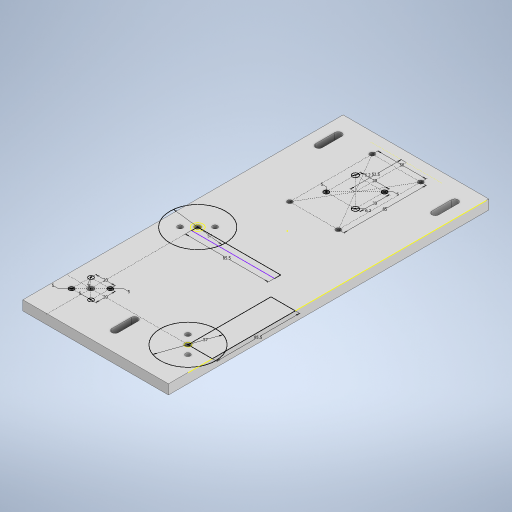
# Autodesk Inventor part: Base
Saved by Autodesk Inventor 2024 (Build 280153000, 153)
## iProperties
Created: 2026-02-25
Part Number: Base
Material: Generic
Document SubType Name: Modeling
Designer: Nathan
Density: 1 g/cm^3
Appearance: Default
Author: Nathan
Autodesk Inventor part; units mm, degrees
ref_plane "YZ Plane" through (0, 0, 0) normal (1, 0, 0) x (0, 1, 0)
ref_plane "XZ Plane" through (0, 0, 0) normal (0, 1, 0) x (-1, 0, 0)
ref_plane "XY Plane" through (0, 0, 0) normal (0, 0, 1) x (1, 0, 0)
sketch "Sketch1" plane through (0, 0, 0) normal (0, 1, 0) x (-1, 0, 0)
  line L0 (90, 130) -> (-90, 130)
  line L1 (-90, 130) -> (-90, -130)
  line L2 (-90, -130) -> (90, -130)
  line L3 (90, -130) -> (90, 130)
  line L4 (90, 130) -> (-90, -130) construction
  line L5 (-90, 130) -> (90, -130) construction
  point P0 (0, 0)
  dimension "d0" = 180
  dimension "d1" = 260
  constraints: 12 end point, 2 midpoint, 2 parallel, 1 horizontal, 1 perpendicular
  measures "d0" distance of L2.end L1.end
  measures "d1" distance of L1.end L0.end
extrude "Extrusion1" add sketch "Sketch1" along normal blind 10
sketch "Sketch2" plane through (0, 10, 0) normal (0, 1, 0) x (1, 0, 0)
  line L0 (90, 130) -> (-90, 130) construction
  line L1 (0, 130) -> (0, 120) construction
  line L2 (0, 130) -> (10, 130) construction
  line L3 (0, 120) -> (0, 70) construction
  line L4 (-37.5, 17.5) -> (37.5, 17.5)
  line L5 (37.5, 17.5) -> (37.5, 122.5)
  line L6 (37.5, 122.5) -> (-37.5, 122.5)
  line L7 (-37.5, 122.5) -> (-37.5, 17.5)
  line L8 (-37.5, 17.5) -> (37.5, 122.5) construction
  line L9 (37.5, 17.5) -> (-37.5, 122.5) construction
  point P0 (0, 0)
  dimension "d4" = 10
  dimension "d6" = 50
  dimension "d7" = 75
  dimension "d8" = 105
  constraints: 18 end point, 3 midpoint, 3 perpendicular, 2 horizontal, 2 parallel, 1 vertical
  measures "d4" distance of L1.start L1.end
  measures "d6" distance of L1.end L3.end
  measures "d7" distance of L6.end L5.end
  measures "d8" distance of L5.end L4.end
extrude "Extrusion2" cut sketch "Sketch2" against normal blind 2
sketch "Sketch3" plane through (0, 8, 0) normal (0, 1, 0) x (1, 0, 0)
  line L0 (-37.5, 122.5) -> (37.5, 122.5) construction
  line L1 (0, 122.5) -> (0, 70) construction
  line L2 (-15, 55) -> (15, 55) construction
  line L3 (15, 55) -> (15, 85) construction
  line L4 (15, 85) -> (-15, 85) construction
  line L5 (-15, 85) -> (-15, 55) construction
  line L6 (-15, 55) -> (15, 85) construction
  line L7 (15, 55) -> (-15, 85) construction
  circle A0 centre (15, 55) radius 3.1
  circle A1 centre (-15, 85) radius 3.1
  line L8 (-25, 27.5) -> (25, 27.5) construction
  line L9 (25, 27.5) -> (25, 112.5) construction
  line L10 (25, 112.5) -> (-25, 112.5) construction
  line L11 (-25, 112.5) -> (-25, 27.5) construction
  line L12 (-25, 27.5) -> (25, 112.5) construction
  line L13 (25, 27.5) -> (-25, 112.5) construction
  circle A2 centre (-15, 55) radius 2.5
  circle A3 centre (15, 85) radius 2.5
  point P0 (0, 0)
  dimension "d11" = 52.5
  dimension "d12" = 30
  dimension "d13" = 30
  dimension "d14" = 6.2
  dimension "d15" = 6.2
  dimension "d19" = 50
  dimension "d20" = 85
  dimension "d175" = 5
  dimension "d176" = 5
  constraints: 26 end point, 5 midpoint, 4 centre point, 4 coincident, 4 parallel, 2 horizontal, 2 perpendicular, 1 vertical
  measures "d11" distance of L1.start L1.end
  measures "d12" distance of L4.end L3.end
  measures "d13" distance of L3.end L2.end
  measures "d14" diameter of A0
  measures "d15" diameter of A1
  measures "d19" distance of L10.end L9.end
  measures "d20" distance of L9.end L8.end
  measures "d175" diameter of A2
  measures "d176" diameter of A3
extrude "Extrusion3" cut sketch "Sketch3" against normal blind 6 contours A2 | A3
hole "Hole1" at (-25, 8, -27.5) at (25, 8, -27.5) at (25, 8, -112.5) at (-25, 8, -112.5) direction (0, -1, 0) diameter 4.917 depth 10 thread size "M6x1" class "6H" standard "ANSI Metric M Profile"
sketch "Sketch6" plane through (0, 10, 0) normal (0, 1, 0) x (1, 0, 0)
  line L0 (90, -130) -> (90, 130) projected
  line L1 (90, -130) -> (-90, -130)
  line L2 (-90, -130) -> (-90, -192.5)
  line L3 (-90, -192.5) -> (90, -192.5)
  line L4 (90, -192.5) -> (90, -130)
  point P0 (0, 0)
  dimension "d101" = 62.5
  constraints: 8 end point, 2 parallel, 1 horizontal, 1 perpendicular
  measures "d101" distance of L2.end L1.end
extrude "Extrusion15" add sketch "Sketch6" against normal blind 10
sketch "Sketch13" plane through (0, 10, 0) normal (0, 1, 0) x (1, 0, 0)
  line L0 (90, -192.5) -> (-90, -192.5) construction
  line L1 (90, -192.5) -> (50, -192.5) construction
  line L2 (50, -192.5) -> (50, -152.5) construction
  line L3 (50, -152.5) -> (90, -152.5) construction
  line L4 (90, -152.5) -> (90, -192.5) construction
  line L5 (-90, 130) -> (-90, -192.5) construction
  line L6 (-90, -192.5) -> (-50, -192.5) construction
  line L7 (-50, -192.5) -> (-50, -42.5) construction
  line L8 (-50, -42.5) -> (-90, -42.5) construction
  line L9 (-90, -42.5) -> (-90, -192.5) construction
  line L10 (32, -170.5) -> (68, -170.5)
  line L11 (68, -170.5) -> (68, -134.5)
  line L12 (68, -134.5) -> (32, -134.5)
  line L13 (32, -134.5) -> (32, -170.5)
  line L14 (32, -170.5) -> (68, -134.5) construction
  line L15 (68, -170.5) -> (32, -134.5) construction
  line L16 (-68, -60.5) -> (-32, -60.5)
  line L17 (-32, -60.5) -> (-32, -24.5)
  line L18 (-32, -24.5) -> (-68, -24.5)
  line L19 (-68, -24.5) -> (-68, -60.5)
  line L20 (-68, -60.5) -> (-32, -24.5) construction
  line L21 (-32, -60.5) -> (-68, -24.5) construction
  point P0 (0, 0)
  dimension "d104" = 40
  dimension "d105" = 40
  dimension "d106" = 40
  dimension "d107" = 150
  dimension "d108" = 36
  dimension "d109" = 36
  dimension "d110" = 36
  dimension "d111" = 36
  constraints: 40 end point, 8 parallel, 4 horizontal, 4 midpoint, 4 perpendicular
  measures "d104" distance of L2.end L3.end
  measures "d105" distance of L1.end L2.end
  measures "d106" distance of L8.end L7.end
  measures "d107" distance of L7.end L6.end
  measures "d108" distance of L12.end L11.end
  measures "d109" distance of L11.end L10.end
  measures "d110" distance of L18.end L17.end
  measures "d111" distance of L17.end L16.end
extrude "Extrusion16" cut sketch "Sketch13" against normal blind 2
sketch "Sketch14" plane through (0, 8, 0) normal (0, 1, 0) x (1, 0, 0)
  line L0 (68, -170.5) -> (32, -170.5) construction
  line L1 (68, -170.5) -> (32, -134.5) construction
  line L2 (68, -134.5) -> (68, -170.5) construction
  line L3 (68, -134.5) -> (32, -170.5) construction
  line L4 (-32, -24.5) -> (-32, -60.5) construction
  line L5 (-32, -60.5) -> (-68, -24.5) construction
  line L6 (-68, -24.5) -> (-32, -24.5) construction
  line L7 (-32, -60.5) -> (-68, -60.5) construction
  line L8 (-32, -24.5) -> (-68, -60.5) construction
  line L9 (50, -152.5) -> (50, -134.5) construction
  line L10 (32, -134.5) -> (68, -134.5) construction
  line L11 (-50, -42.5) -> (-50, -24.5) construction
  line L12 (41, -161.5) -> (59, -161.5) construction
  line L13 (59, -161.5) -> (59, -143.5) construction
  line L14 (59, -143.5) -> (41, -143.5) construction
  line L15 (41, -143.5) -> (41, -161.5) construction
  line L16 (41, -161.5) -> (59, -143.5) construction
  line L17 (59, -161.5) -> (41, -143.5) construction
  line L18 (-59, -51.5) -> (-41, -51.5) construction
  line L19 (-41, -51.5) -> (-41, -33.5) construction
  line L20 (-41, -33.5) -> (-59, -33.5) construction
  line L21 (-59, -33.5) -> (-59, -51.5) construction
  line L22 (-59, -51.5) -> (-41, -33.5) construction
  line L23 (-41, -51.5) -> (-59, -33.5) construction
  circle A0 centre (59, -161.5) radius 2.5
  circle A1 centre (41, -143.5) radius 2.5
  circle A2 centre (-59, -51.5) radius 2.5
  circle A3 centre (-41, -33.5) radius 2.5
  point P0 (0, 0)
  dimension "d121" = 18
  dimension "d122" = 18
  dimension "d123" = 18
  dimension "d124" = 18
  dimension "d125" = 5
  dimension "d126" = 5
  dimension "d127" = 5
  dimension "d128" = 5
  constraints: 36 end point, 8 midpoint, 4 centre point, 4 coincident, 4 parallel, 3 perpendicular, 2 horizontal
  measures "d121" distance of L14.end L13.end
  measures "d122" distance of L13.end L12.end
  measures "d123" distance of L20.end L19.end
  measures "d124" distance of L19.end L18.end
  measures "d125" diameter of A0
  measures "d126" diameter of A1
  measures "d127" diameter of A2
  measures "d128" diameter of A3
sketch "Sketch15" plane through (0, 0, 0) normal (0, -1, 0) x (1, 0, 0)
  line L0 (68, 134.5) -> (68, 170.5) construction
  line L1 (68, 170.5) -> (32, 134.5) construction
  line L2 (32, 134.5) -> (68, 134.5) construction
  line L3 (68, 134.5) -> (32, 170.5) construction
  line L4 (32, 170.5) -> (50, 152.5) construction
  line L5 (-32, 24.5) -> (-32, 60.5) construction
  line L6 (-32, 60.5) -> (-68, 24.5) construction
  line L7 (-68, 24.5) -> (-32, 24.5) construction
  line L8 (-32, 24.5) -> (-68, 60.5) construction
  line L9 (-68, 60.5) -> (-50, 42.5) construction
  point P0 (0, 0)
  constraints: 15 end point, 2 midpoint, 2 perpendicular
extrude "Extrusion17" cut sketch "Sketch14" against normal blind 6
sketch "Sketch16" plane through (0, 10, 0) normal (0, 1, 0) x (1, 0, 0)
  line L0 (32, -170.5) -> (32, -134.5) construction
  line L1 (32, -134.5) -> (-90, -134.5) construction
  line L2 (-90, 130) -> (-90, -192.5) construction
  line L3 (32, -170.5) -> (-90, -170.5) construction
  line L4 (-32, -60.5) -> (-68, -60.5) construction
  line L5 (-32, -60.5) -> (-32, -134.5) construction
  line L6 (-32, -134.5) -> (-63, -134.5)
  line L7 (-63, -134.5) -> (-63, -165.5)
  line L8 (-63, -165.5) -> (-32, -165.5)
  line L9 (-32, -165.5) -> (-32, -134.5)
  point P0 (0, 0)
  dimension "d140" = 31
  dimension "d141" = 31
  constraints: 14 end point, 3 horizontal, 2 parallel, 2 point on line, 1 perpendicular, 1 vertical
  measures "d140" distance of L8.end L7.end
  measures "d141" distance of L7.end L6.end
extrude "Extrusion18" cut sketch "Sketch16" against normal blind 2
sketch "Sketch18" plane through (0, 0, 0) normal (0, -1, 0) x (1, 0, 0)
  line L0 (-90, 192.5) -> (90, 192.5) projected
  line L1 (-90, -130) -> (-90, 192.5) projected
  line L2 (90, 192.5) -> (-90, 192.5)
  line L3 (-90, 192.5) -> (-90, -130)
  line L4 (-90, -130) -> (90, -130)
  line L5 (90, -130) -> (90, 192.5)
  point P0 (0, 0)
  constraints: 8 end point, 2 parallel, 1 horizontal, 1 perpendicular
extrude "Extrusion20" add sketch "Sketch18" along normal blind 2
sketch "Sketch19" plane through (0, -2, 0) normal (0, -1, 0) x (1, 0, 0)
  circle A0 centre (50, 152.5) radius 2.4585 construction
  circle A1 centre (-50, 42.5) radius 2.4585 construction
  line L0 (50, 152.5) -> (-50, 42.5) construction
  line L1 (-32, 165.5) -> (-63, 165.5) construction
  line L2 (-32, 134.5) -> (-32, 165.5) construction
  line L3 (-63, 165.5) -> (-32, 134.5) construction
  line L4 (-63, 134.5) -> (-32, 134.5) construction
  line L5 (-63, 134.5) -> (-32, 165.5) construction
  line L6 (-47.5, 150) -> (-32, 150) construction
  point P0 (0, 0)
  constraints: 8 end point, 2 midpoint
hole "Hole6" at (-50, -2, 42.5) at (50, -2, 152.5) direction (0, 1, 0) diameter 6.1 end through all countersink diameter 11 countersink angle 90 clearance for "Countersunk Flat Head Screw ISO 2009/7046" size "M6" standard "ISO"
sketch "Sketch20" plane through (0, 10, 0) normal (0, 1, 0) x (1, 0, 0)
  line L0 (-90, 130) -> (90, 130) construction
  line L1 (-90, -192.5) -> (-90, 130) construction
  line L2 (90, 130) -> (-90, 130) construction
  line L3 (-90, 130) -> (-90, -192.5) construction
  line L4 (-90, -192.5) -> (90, -192.5) construction
  line L5 (90, -192.5) -> (90, 130) construction
  line L6 (-90, -192.5) -> (-75, -192.5)
  line L7 (-75, -177.5) -> (-75, 130)
  line L8 (-75, 130) -> (-90, 130)
  line L9 (-90, 130) -> (-90, -192.5)
  line L10 (90, 130) -> (75, 130)
  line L11 (75, 130) -> (75, -177.5)
  line L12 (75, -192.5) -> (90, -192.5)
  line L13 (90, -192.5) -> (90, 130)
  line L14 (90, -192.5) -> (-90, -192.5)
  line L15 (-90, -192.5) -> (-90, -177.5)
  line L16 (-75, -177.5) -> (75, -177.5)
  line L17 (90, -177.5) -> (90, -192.5)
  point P0 (0, 0)
  dimension "d166" = 180
  dimension "d167" = 15
  dimension "d168" = 15
  dimension "d169" = 15
  constraints: 32 end point, 8 parallel, 4 horizontal, 4 perpendicular, 3 point on line
  measures "d166" distance of L4.end L1.start
  measures "d167" distance of L8.end L7.end
  measures "d168" distance of L12.end L12.start
  measures "d169" distance of L14.end L15.end
extrude "Extrusion21" cut sketch "Sketch20" against normal through all
sketch "Sketch21" plane through (0, 10, 0) normal (0, 1, 0) x (1, 0, 0)
  line L0 (-75, -177.5) -> (-75, 130) projected
  line L1 (75, 130) -> (75, -177.5) projected
  line L2 (-75, -177.5) -> (75, -177.5)
  line L3 (75, -177.5) -> (75, 130)
  line L4 (75, 130) -> (-75, 130)
  line L5 (-75, 130) -> (-75, -177.5)
  point P0 (0, 0)
  constraints: 8 end point, 2 parallel, 1 horizontal, 1 perpendicular
extrude "Extrusion22" cut sketch "Sketch21" against normal blind 2
sketch "Sketch22" plane through (0, 8, 0) normal (0, 1, 0) x (1, 0, 0)
  circle A0 centre (-50, -42.5) radius 3.05 projected
  circle A1 centre (-50, -42.5) radius 28.5
  circle A2 centre (50, -152.5) radius 3.05 projected
  circle A3 centre (50, -152.5) radius 28.5
  line L0 (75, 130) -> (75, -177.5) projected
  line L1 (50, -152.5) -> (75, -152.5)
  line L2 (75, -152.5) -> (75, -67)
  line L3 (75, -67) -> (50, -67)
  line L4 (50, -67) -> (50, -152.5)
  circle A4 centre (-50, -42.5) radius 5.5 projected
  line L5 (-50, -42.5) -> (35.5, -42.5)
  line L6 (35.5, -42.5) -> (35.5, -48.8)
  line L7 (35.5, -48.8) -> (-50, -48.8)
  line L8 (-50, -48.8) -> (-50, -42.5)
  point P0 (0, 0)
  dimension "d182" = 57
  dimension "d183" = 57
  dimension "d184" = 85.5
  dimension "d185" = 85.5
  constraints: 16 end point, 4 parallel, 2 centre point, 2 coincident, 2 horizontal, 2 perpendicular, 1 point on line
  measures "d182" diameter of A1
  measures "d183" diameter of A3
  measures "d184" distance of L2.end L1.end
  measures "d185" distance of L6.end L7.end
sketch "Sketch23" plane through (0, 8, 0) normal (0, 1, 0) x (1, 0, 0)
  line L0 (75, 130) -> (75, -177.5) projected
  line L1 (-75, -177.5) -> (-75, 130) projected
  line L2 (75, 130) -> (-75, 130)
  line L3 (-75, 130) -> (-75, -177.5)
  line L4 (-75, -177.5) -> (75, -177.5)
  line L5 (75, -177.5) -> (75, 130)
  line L6 (-75, 130) -> (75, 130) projected
  line L7 (75, 130) -> (-75, 130)
  line L8 (-75, 130) -> (-75, 132.5)
  line L9 (-75, 132.5) -> (75, 132.5)
  line L10 (75, 132.5) -> (75, 130)
  line L11 (-75, -177.5) -> (75, -177.5)
  line L12 (75, -177.5) -> (75, -197.5)
  line L13 (75, -197.5) -> (-75, -197.5)
  line L14 (-75, -197.5) -> (-75, -177.5)
  point P0 (0, 0)
  dimension "d186" = 2.5
  dimension "d187" = 20
  constraints: 24 end point, 6 parallel, 3 horizontal, 3 perpendicular
  measures "d186" distance of L7.end L8.end
  measures "d187" distance of L11.end L12.end
extrude "Extrusion23" add sketch "Sketch23" against normal blind 10 contours L2 L8 L9 L10 | L12 L13 L14 L4
sketch "Sketch24" plane through (0, 8, 0) normal (0, 1, 0) x (1, 0, 0)
  circle A0 centre (50, -152.5) radius 3.05 construction
  line L0 (50, -152.5) -> (-74.625, -152.5) construction
  circle A1 centre (-50, -42.5) radius 3.05 construction
  line L1 (-50, -42.5) -> (-50, -199.1809) construction
  line L2 (-60, -162.5) -> (-40, -162.5) construction
  line L3 (-40, -162.5) -> (-40, -142.5) construction
  line L4 (-40, -142.5) -> (-60, -142.5) construction
  line L5 (-60, -142.5) -> (-60, -162.5) construction
  line L6 (-60, -162.5) -> (-40, -142.5) construction
  line L7 (-40, -162.5) -> (-60, -142.5) construction
  circle A2 centre (-60, -162.5) radius 2.5
  circle A3 centre (-40, -142.5) radius 2.5
  circle A4 centre (-40, -162.5) radius 2.5
  circle A5 centre (-60, -142.5) radius 2.5
  point P0 (0, 0)
  point P1 (-50, -152.5)
  dimension "d190" = 20
  dimension "d191" = 20
  dimension "d192" = 5
  dimension "d193" = 5
  dimension "d221" = 5
  dimension "d222" = 5
  constraints: 16 end point, 4 centre point, 4 coincident, 2 horizontal, 2 midpoint, 2 parallel, 2 perpendicular, 2 point on line
  measures "d190" distance of L4.end L3.end
  measures "d191" distance of L3.end L2.end
  measures "d192" diameter of A2
  measures "d193" diameter of A3
  measures "d221" diameter of A4
  measures "d222" diameter of A5
extrude "Extrusion24" cut sketch "Sketch24" against normal blind 6 contours A2 | A3
sketch "Sketch25" plane through (0, -2, 0) normal (0, -1, 0) x (1, 0, 0)
  circle A0 centre (50, 152.5) radius 3.05 construction
  line L0 (50, 152.5) -> (-75, 152.5) construction
  line L1 (-75, 197.5) -> (-75, -132.5) construction
  circle A1 centre (-50, 42.5) radius 3.05 construction
  line L2 (-50, 42.5) -> (-50, 197.5) construction
  line L3 (75, 197.5) -> (-75, 197.5) construction
  circle A2 centre (-50, 152.5) radius 7.5 construction
  point P0 (0, 0)
  dimension "d213" = 15
  constraints: 4 end point, 4 point on line, 1 centre point, 1 horizontal, 1 perpendicular
  measures "d213" diameter of A2
hole "Hole10" at (-50, -2, 152.5) direction (0, 1, 0) diameter 6.1 end through all countersink diameter 11 countersink angle 90 clearance for "Countersunk Flat Head Screw ISO 2009/7046" size "M6" standard "ISO"
sketch "Sketch26" plane through (0, 8, 0) normal (0, 1, 0) x (1, 0, 0)
  line L0 (-75, -197.5) -> (-75, 132.5) construction
  line L1 (-75, 132.5) -> (-75, -32.5) construction
  line L2 (-75, -32.5) -> (0, -32.5) construction
  line L3 (75, -172.5) -> (-75, -172.5) construction
  line L4 (-75, -172.5) -> (-75, 107.5) construction
  line L5 (-75, 107.5) -> (75, 107.5) construction
  line L6 (75, 107.5) -> (75, -172.5) construction
  line L7 (75, -172.5) -> (-75, 107.5) construction
  line L8 (-75, -172.5) -> (75, 107.5) construction
  line L9 (0, -172.5) -> (0, -32.5) construction
  line L10 (0, -172.5) -> (0, -177.5) construction
  line L11 (0, 107.5) -> (-60, 107.5) construction
  line L12 (0, 107.5) -> (60, 107.5) construction
  line L13 (-60, 107.5) -> (-60, 112.5) construction
  line L14 (60, 107.5) -> (60, 112.5) construction
  line L15 (0, -177.5) -> (0, -157.5) construction
  line L16 (3.5, -177.5) -> (3.5, -157.5)
  line L17 (-3.5, -157.5) -> (-3.5, -177.5)
  arc A0 (-3.5, -177.5) -> (3.5, -177.5) centre (0, -177.5) ccw
  arc A1 (3.5, -157.5) -> (-3.5, -157.5) centre (0, -157.5) ccw
  line L18 (-60, 112.5) -> (-60, 92.5) construction
  line L19 (-63.5, 112.5) -> (-63.5, 92.5)
  line L20 (-56.5, 92.5) -> (-56.5, 112.5)
  arc A2 (-56.5, 112.5) -> (-63.5, 112.5) centre (-60, 112.5) ccw
  arc A3 (-63.5, 92.5) -> (-56.5, 92.5) centre (-60, 92.5) ccw
  line L21 (60, 112.5) -> (60, 92.5) construction
  line L22 (56.5, 112.5) -> (56.5, 92.5)
  line L23 (63.5, 92.5) -> (63.5, 112.5)
  arc A4 (63.5, 112.5) -> (56.5, 112.5) centre (60, 112.5) ccw
  arc A5 (56.5, 92.5) -> (63.5, 92.5) centre (60, 92.5) ccw
  point P0 (0, 0)
  point P1 (0, -167.5)
  point P2 (-60, 102.5)
  point P3 (60, 102.5)
  dimension "d223" = 165
  dimension "d224" = 280
  dimension "d225" = 5
  dimension "d226" = 60
  dimension "d227" = 60
  dimension "d228" = 5
  dimension "d229" = 5
  dimension "d230" = 20
  dimension "d231" = 7
  dimension "d232" = 20
  dimension "d233" = 7
  dimension "d234" = 20
  dimension "d235" = 7
  constraints: 52 end point, 12 point on circle, 12 tangent, 7 midpoint, 6 centre point, 5 parallel, 5 vertical, 4 perpendicular, 4 point on line, 1 horizontal
  measures "d223" distance of L0.end L1.end
  measures "d224" distance of L3.end L4.end
  measures "d225" distance of L9.start L10.end
  measures "d226" distance of L11.start L11.end
  measures "d227" distance of L11.start L12.end
  measures "d228" distance of L11.end L13.end
  measures "d229" distance of L12.end L14.end
  measures "d230" distance of L10.end L15.end
  measures "d231" diameter of A1
  measures "d232" distance of L13.end L18.end
  measures "d233" diameter of A3
  measures "d234" distance of L14.end L21.end
  measures "d235" diameter of A5
extrude "Extrusion25" cut sketch "Sketch26" against normal through all
body "Solid1"
